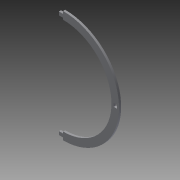
# Autodesk Inventor part: TopfemaleHoopSection_v1
Saved by Autodesk Inventor 2013 (Build 170138000, 138)
## iProperties
Created: 2013-01-17
Part Number: TopfemaleHoopSection_v1
Material: Generic
Document SubType Name: Modeling
Designer: twsass
Density: 1 g/cm^3
Author: twsass
Autodesk Inventor part; units mm, degrees
ref_plane "YZ Plane" through (0, 0, 0) normal (1, 0, 0) x (0, 1, 0)
ref_plane "XZ Plane" through (0, 0, 0) normal (0, 1, 0) x (-1, 0, 0)
ref_plane "XY Plane" through (0, 0, 0) normal (0, 0, 1) x (1, 0, 0)
sketch "Sketch1" plane through (0, 0, 0) normal (0, 0, 1) x (1, 0, 0)
  circle A0 centre (0, 0) radius 146.05
  circle A1 centre (0, 0) radius 168.91
  line L0 (0, -146.05) -> (0, -168.91)
  line L1 (0, 168.91) -> (0, 146.05)
  line L2 (0, 168.91) -> (0, -168.91) construction
  circle A2 centre (-157.48, 0) radius 3.175
  line L3 (0, 146.05) -> (0, 151.13)
  line L4 (0, 151.13) -> (-12.7, 151.13)
  line L5 (-12.7, 151.13) -> (-12.7, 161.29)
  line L6 (-12.7, 161.29) -> (0, 161.29)
  line L7 (0, 161.29) -> (0, 151.13)
  line L8 (0, -146.05) -> (0, -151.13)
  line L9 (0, -151.13) -> (-12.7, -151.13)
  line L10 (-12.7, -151.13) -> (-12.7, -161.29)
  line L11 (-12.7, -161.29) -> (0, -161.29)
  line L12 (0, -151.13) -> (0, -161.29)
  line L13 (157.48, 0) -> (157.48, 5.08)
  line L14 (157.48, 5.08) -> (162.2425, 5.08)
  line L15 (162.2425, 5.08) -> (162.2425, -5.08)
  line L16 (162.2425, -5.08) -> (152.7175, -5.08)
  line L17 (152.7175, -5.08) -> (152.7175, 5.08)
  line L18 (152.7175, 5.08) -> (157.48, 5.08)
  dimension "d51" = 292.1
  dimension "d52" = 337.82
  dimension "d55" = 5.08
  dimension "d56" = 12.7
  dimension "d57" = 10.16
  dimension "d58" = 5.08
  dimension "d59" = 12.7
  dimension "d60" = 10.16
  dimension "d63" = 5.08
  dimension "d64" = 4.7625
  dimension "d65" = 10.16
  dimension "d66" = 9.525
  dimension "d67" = 157.48
  constraints: 38 end point, 6 parallel, 5 collinear, 5 perpendicular, 5 point on circle, 4 point on line, 3 centre point, 1 coincident, 1 vertical
  measures "d51" diameter of A0
  measures "d52" diameter of A1
  measures "d55" distance of L1.end L3.end
  measures "d56" distance of L3.end L4.end
  measures "d57" distance of L4.end L5.end
  measures "d58" distance of L0.start L8.end
  measures "d59" distance of L8.end L9.end
  measures "d60" distance of L9.end L10.end
  measures "d63" distance of L13.start L13.end
  measures "d64" distance of L13.end L14.end
  measures "d65" distance of L14.end L15.end
  measures "d66" distance of L15.end L16.end
  measures "d67" distance of A0.centre L13.start
extrude "Extrusion12" add sketch "Sketch1" along normal blind 6.35 contours A0 L1 A1 L0 | L4 L5 L6 L1 | L0 L11 L10 L9
body "Solid5"
